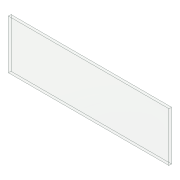
# Autodesk Inventor part: Sharp 2Y0A02 Case Screen
Saved by Autodesk Inventor 2018.3 (Build 223284000, 284)
## iProperties
Created: 2019-01-03
Part Number: Sharp 2Y0A02 Case Screen
Material: Glass
Document SubType Name: Modeling
Designer: aye06091
Mass: 1.09829 g
Surface Area: 14.1484 cm^2
Volume: 0.503804 cm^3
Density: 2.18 g/cm^3
Appearance: Clear
Author: aye06091
Autodesk Inventor part; units mm, degrees
ref_plane "YZ Plane" through (0, 0, 0) normal (1, 0, 0) x (0, 1, 0)
ref_plane "XZ Plane" through (0, 0, 0) normal (0, 1, 0) x (-1, 0, 0)
ref_plane "XY Plane" through (0, 0, 0) normal (0, 0, 1) x (1, 0, 0)
sketch "Sketch1" plane through (0, 0, 0) normal (0, 0, 1) x (1, 0, 0)
  line L0 (0, 0) -> (46.482, 0)
  line L1 (46.482, 0) -> (46.482, -14.224)
  line L2 (46.482, -14.224) -> (0, -14.224)
  line L3 (0, -14.224) -> (0, 0)
  dimension "d0" = 46.482
  dimension "d1" = 14.224
  constraints: 8 end point, 2 parallel, 1 horizontal, 1 perpendicular
  measures "d0" distance of L1.end L2.end
  measures "d1" distance of L0.end L1.end
extrude "Extrusion1" add sketch "Sketch1" against normal blind 0.762
body "Solid1"
